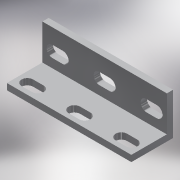
# Autodesk Inventor part: L bracket triple
Saved by Autodesk Inventor 2020.3 (Build 243373000, 373)
## iProperties
Created: 2016-04-18
Part Number: L bracket triple
Material: Aluminum
Document SubType Name: Modeling
Designer: Ben
Density: 2.7 g/cm^3
Appearance: Aluminum - Dark
Author: Ben
Autodesk Inventor part; units mm, degrees
ref_plane "YZ Plane" through (0, 0, 0) normal (1, 0, 0) x (0, 1, 0)
ref_plane "XZ Plane" through (0, 0, 0) normal (0, 1, 0) x (-1, 0, 0)
ref_plane "XY Plane" through (0, 0, 0) normal (0, 0, 1) x (1, 0, 0)
sketch "Sketch1" plane through (0, 0, 0) normal (0, 0, 1) x (1, 0, 0)
  line L0 (-29.8, 10) -> (29.8, 10)
  line L1 (29.8, 10) -> (29.8, -10)
  line L2 (29.8, -10) -> (-29.8, -10)
  line L3 (-29.8, -10) -> (-29.8, 10)
  line L4 (0, 10) -> (0, -10) construction
  line L5 (-29.8, 0) -> (29.8, 0) construction
  line L6 (-2.5, 0) -> (2.5, 0) construction
  line L7 (-2.5, -2.75) -> (2.5, -2.75)
  line L8 (2.5, 2.75) -> (-2.5, 2.75)
  arc A0 (-2.5, 2.75) -> (-2.5, -2.75) centre (-2.5, 0) ccw
  arc A1 (2.5, -2.75) -> (2.5, 2.75) centre (2.5, 0) ccw
  line L9 (-25, 0) -> (-20, 0) construction
  line L10 (-25, -2.75) -> (-20, -2.75)
  line L11 (-20, 2.75) -> (-25, 2.75)
  arc A2 (-25, 2.75) -> (-25, -2.75) centre (-25, 0) ccw
  arc A3 (-20, -2.75) -> (-20, 2.75) centre (-20, 0) ccw
  line L12 (20, 0) -> (25, 0) construction
  line L13 (20, -2.75) -> (25, -2.75)
  line L14 (25, 2.75) -> (20, 2.75)
  arc A4 (20, 2.75) -> (20, -2.75) centre (20, 0) ccw
  arc A5 (25, -2.75) -> (25, 2.75) centre (25, 0) ccw
  point P0 (0, 0)
  point P1 (0, 0)
  point P2 (0, 0)
  point P3 (-22.5, 0)
  point P4 (22.5, 0)
  dimension "d0" = 20
  dimension "d1" = 59.6
  dimension "d17" = 5
  dimension "d18" = 5.5
  dimension "d19" = 5.5
  dimension "d20" = 5
  dimension "d21" = 5.5
  dimension "d22" = 5
  dimension "d23" = 22.5
  dimension "d24" = 22.5
  constraints: 34 end point, 12 point on circle, 12 tangent, 8 midpoint, 6 centre point, 5 parallel, 1 coincident, 1 horizontal, 1 perpendicular, 11 other
  measures "d0" distance of L2.end L0.start
  measures "d1" distance of L0.start L0.end
  measures "d17" distance of L6.start L6.end
  measures "d18" diameter of A1
  measures "d19" diameter of A3
  measures "d20" distance of L12.start L12.end
  measures "d21" diameter of A5
  measures "d22" distance of L9.end L9.start
  measures "d23" distance from line of L4 point (-22.5, 0)
  measures "d24" distance from line of L4 point (22.5, 0)
extrude "Extrusion1" add sketch "Sketch1" along normal blind 3
sketch "Sketch2" plane through (0, 0, 3) normal (0, 0, 1) x (1, 0, 0)
  line L0 (29.8, -10) -> (29.8, 10) projected
  line L1 (-29.8, -10) -> (29.8, -10)
  line L2 (29.8, -10) -> (29.8, -7)
  line L3 (29.8, -7) -> (-29.8, -7)
  line L4 (-29.8, -7) -> (-29.8, -10)
  point P0 (0, 0)
  dimension "d7" = 3
  constraints: 8 end point, 2 parallel, 1 horizontal, 1 perpendicular, 1 point on line
  measures "d7" distance of L1.end L2.end
extrude "Extrusion2" add sketch "Sketch2" along normal blind 17
sketch "Sketch3" plane through (-29.8, -7, 3) normal (0, 1, 0) x (1, 0, 0)
  line L0 (0, 0) -> (0, -17) projected
  line L1 (59.6, -17) -> (0, -17) projected
  line L2 (59.6, 0) -> (59.6, -17) projected
  line L3 (0, -12) -> (59.6, -12) construction
  line L4 (0, 0) -> (59.6, 0) projected
  line L5 (29.8, 0) -> (29.8, -17) construction
  line L6 (27.3, -12) -> (32.3, -12) construction
  line L7 (27.3, -14.75) -> (32.3, -14.75)
  line L8 (32.3, -9.25) -> (27.3, -9.25)
  arc A0 (27.3, -9.25) -> (27.3, -14.75) centre (27.3, -12) ccw
  arc A1 (32.3, -14.75) -> (32.3, -9.25) centre (32.3, -12) ccw
  line L9 (4.8, -12) -> (9.8, -12) construction
  line L10 (4.8, -14.75) -> (9.8, -14.75)
  line L11 (9.8, -9.25) -> (4.8, -9.25)
  arc A2 (4.8, -9.25) -> (4.8, -14.75) centre (4.8, -12) ccw
  arc A3 (9.8, -14.75) -> (9.8, -9.25) centre (9.8, -12) ccw
  line L12 (49.8, -12) -> (54.8, -12) construction
  line L13 (49.8, -14.75) -> (54.8, -14.75)
  line L14 (54.8, -9.25) -> (49.8, -9.25)
  arc A4 (49.8, -9.25) -> (49.8, -14.75) centre (49.8, -12) ccw
  arc A5 (54.8, -14.75) -> (54.8, -9.25) centre (54.8, -12) ccw
  point P0 (29.8, 3)
  point P1 (29.8, -12)
  point P2 (29.8, -12)
  point P3 (7.3, -12)
  point P4 (52.3, -12)
  dimension "d12" = 5
  dimension "d25" = 5
  dimension "d26" = 5.5
  dimension "d27" = 5
  dimension "d28" = 5.5
  dimension "d29" = 5
  dimension "d30" = 5.5
  dimension "d31" = 22.5
  dimension "d32" = 22.5
  constraints: 26 end point, 12 point on circle, 12 tangent, 6 centre point, 5 midpoint, 3 parallel, 2 point on line, 1 coincident, 1 vertical, 10 other
  measures "d25" distance of L6.start L6.end
  measures "d26" diameter of A1
  measures "d27" distance of L9.start L9.end
  measures "d28" diameter of A3
  measures "d29" distance of L12.start L12.end
  measures "d30" diameter of A5
  measures "d31" distance of point (29.8, -12) point (7.3, -12)
  measures "d32" distance of point (52.3, -12) point (29.8, -12)
extrude "Extrusion3" cut sketch "Sketch3" against normal up to surface (3 mm away) contours A0 L8 A1 L7 | A2 L11 A3 L10 | A4 L14 A5 L13
body "Solid1"
